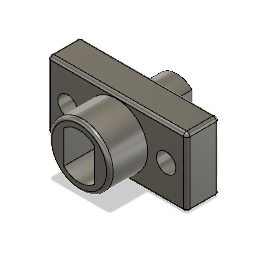
3d platform holder v1 v3 (Autodesk Fusion 360 design; units mm, degrees)
Autodesk Fusion 360 part; units mm, degrees
sketch "Sketch1" plane through (0, 0, 0) normal (0, 0, 1) x (1, 0, 0)
  circle A0 centre (0, 0) radius 4.7625
  dimension "d1" = 9.525
  measures "d1" diameter of A0
extrude "Extrude1" add sketch "Sketch1" along normal blind 11.43 makes body 1
sketch "Sketch2" plane through (0, 0, 11.43) normal (0, 0, 1) x (1, 0, 0)
  circle A0 centre (0, 0) radius 4.7625
  line L0 (-2.3876, 2.5527) -> (-2.3876, -2.5527)
  line L1 (2.3876, -2.5527) -> (2.3876, 2.5527)
  line L2 (2.3876, 2.5527) -> (-2.3876, -2.5527) construction
  line L3 (-2.3876, 2.5527) -> (2.3876, -2.5527) construction
  arc A1 (2.3876, 2.5527) -> (-2.3876, 2.5527) centre (0, 0.0915) ccw
  arc A2 (-2.3876, -2.5527) -> (2.3876, -2.5527) centre (0, -0.0771) ccw
  dimension "d4" = 5.1054
  dimension "d5" = 4.7752
  dimension "d6" = 3.429
  dimension "d7" = 3.4394
  measures "d6" radius of A1
  measures "d7" radius of A2
extrude "Extrude2" cut sketch "Sketch2" against normal blind 5.1562 contours L0 L1 A1 A2 bodies 1
extrude "Extrude3" cut 1 faces at (0.58, -0.1002, 0) along direction (0, 0, 1) blind 3.048 on bodies 1 bodies 1
sketch "Sketch3" plane through (0, 0, 3.048) normal (0, 0, -1) x (-1, 0, 0)
  circle A0 centre (0, 0) radius 4.7625
  line L0 (-10.795, 5.334) -> (10.795, 5.334)
  line L1 (10.795, 5.334) -> (10.795, -5.334)
  line L2 (10.795, -5.334) -> (-10.795, -5.334)
  line L3 (-10.795, -5.334) -> (-10.795, 5.334)
  line L4 (-10.795, 5.334) -> (10.795, -5.334) construction
  line L5 (10.795, 5.334) -> (-10.795, -5.334) construction
  dimension "d12" = 21.59
  dimension "d13" = 10.668
extrude "Extrude5" add sketch "Sketch3" against normal blind 2.54 bodies 1
extrude "Extrude4" add sketch "Sketch3" along normal blind 2.54 contours A0 | L0 L1 L2 L3 bodies 1
sketch "Sketch4" plane through (0, 0, 0.508) normal (0, 0, -1) x (-1, 0, 0)
  line L0 (-10.795, -5.334) -> (10.795, -5.334)
  line L1 (10.795, -5.334) -> (10.795, 5.334)
  line L2 (10.795, 5.334) -> (-10.795, 5.334)
  line L3 (-10.795, 5.334) -> (-10.795, -5.334)
  circle A0 centre (0, 0) radius 1.5
  circle A1 centre (-7.62, 0) radius 1.5
  circle A2 centre (7.62, 0) radius 1.5
  dimension "d18" = 3
  dimension "d19" = 3
  dimension "d20" = 3
  measures "d18" diameter of A2
  measures "d19" diameter of A0
  measures "d20" diameter of A1
extrude "Extrude6" cut sketch "Sketch4" against normal blind 13.97 contours A0 | A1 | A2 bodies 1
sketch "Sketch5" plane through (0, 0, 0.508) normal (0, 0, -1) x (-1, 0, 0)
  circle A0 centre (-7.62, 0) radius 1.5
  circle A1 centre (0, 0) radius 1.5
  circle A2 centre (7.62, 0) radius 1.5
  line L0 (-10.795, -5.334) -> (10.795, -5.334)
  line L1 (10.795, -5.334) -> (10.795, 5.334)
  line L2 (10.795, 5.334) -> (-10.795, 5.334)
  line L3 (-10.795, 5.334) -> (-10.795, -5.334)
  line L4 (-2.3876, -2.5527) -> (-2.3876, 2.5527)
  line L5 (-2.3876, 2.5527) -> (-2.3876, -2.5527)
  line L6 (2.3876, 2.5527) -> (2.3876, -2.5527)
  arc A3 (2.3876, 2.5527) -> (-2.3876, 2.5527) centre (0, 0.0915) ccw
  arc A4 (-2.3876, -2.5527) -> (2.3876, -2.5527) centre (0, -0.0771) ccw
extrude "Extrude7" add sketch "Sketch5" along normal blind 4.191 contours L4 L5 L6 A3 A4 bodies 1
fillet "Fillet1" radius 0.508 13 edges at (-10.795, -5.334, 3.048) (-10.795, 5.334, 3.048) (10.795, 5.334, 3.048) (10.795, -5.334, 3.048) (10.795, 0, 5.588) (10.795, 0, 0.508) (0, 5.334, 0.508) (0, 5.334, 5.588) (-10.795, 0, 5.588) (-10.795, 0, 0.508) (0, -5.334, 5.588) (0, -5.334, 0.508) (-4.4402, -1.7222, 11.43) on bodies 1
sketch "Sketch6" plane through (0, 0, 0.508) normal (0, 0, -1) x (-1, 0, 0)
  circle A0 centre (7.62, 0) radius 1.5
  circle A1 centre (-7.62, 0) radius 1.5
  line L0 (2.3876, 2.5527) -> (2.3876, -2.5527)
  arc A2 (-2.3876, -2.5527) -> (2.3876, -2.5527) centre (0, -0.0771) ccw
  line L1 (-2.3876, -2.5527) -> (-2.3876, 2.5527)
  arc A3 (2.3876, 2.5527) -> (-2.3876, 2.5527) centre (0, 0.0915) ccw
  line L2 (10.287, -4.826) -> (10.287, 4.826)
  line L3 (10.287, 4.826) -> (-10.287, 4.826)
  line L4 (-10.287, 4.826) -> (-10.287, -4.826)
  line L5 (-10.287, -4.826) -> (10.287, -4.826)
  circle A4 centre (0, 0.0915) radius 17.2202
  circle A5 centre (-7.62, 0) radius 1.5
  line L6 (-2.3876, 2.5527) -> (-2.3876, -2.5527)
  arc A6 (2.3876, 2.5527) -> (-2.3876, 2.5527) centre (0, 0.0915) ccw
  line L7 (2.3876, -2.5527) -> (2.3876, 2.5527)
  arc A7 (-2.3876, -2.5527) -> (2.3876, -2.5527) centre (0, -0.0771) ccw
  circle A8 centre (7.62, 0) radius 1.5
extrude "Extrude8" add sketch "Sketch6" along normal blind 3.81 separate body contours L2 L3 L4 L5 | A4 makes body 2
hidden bodies 2
